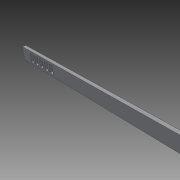
# Autodesk Inventor part: front_pane_middle
Saved by Autodesk Inventor 2014 (Build 180170000, 170)
## iProperties
Created: 2014-03-23
Part Number: front_pane_middle
Material: Generic
Document SubType Name: Modeling
Designer: buben
Density: 1 g/cm^3
Appearance: Default
Author: buben
Autodesk Inventor part; units mm, degrees
ref_plane "YZ Plane" through (0, 0, 0) normal (1, 0, 0) x (0, 1, 0)
ref_plane "XZ Plane" through (0, 0, 0) normal (0, 1, 0) x (-1, 0, 0)
ref_plane "XY Plane" through (0, 0, 0) normal (0, 0, 1) x (1, 0, 0)
sketch "Sketch1" plane through (0, 0, 0) normal (0, 1, 0) x (-1, 0, 0)
  line L0 (0, 0) -> (-300, 0)
  line L1 (-300, 0) -> (-300, -23.685)
  line L2 (-300, -23.685) -> (0, -23.685)
  line L3 (0, -23.685) -> (0, 0)
  dimension "d0" = 300
  dimension "d1" = 23.685
  constraints: 8 end point, 2 parallel, 1 horizontal, 1 perpendicular
  measures "d0" distance of L0.start L0.end
  measures "d1" distance of L2.end L0.start
extrude "Extrusion1" add sketch "Sketch1" along normal blind 6.5
sketch "Sketch2" plane through (0, 6.5, 0) normal (0, 1, 0) x (1, 0, 0)
  line L0 (0, 23.685) -> (0, 0) projected
  line L1 (21, 19.3425) -> (27, 19.3425)
  line L2 (28, 18.3425) -> (28, 5.3425)
  line L3 (27, 4.3425) -> (21, 4.3425)
  line L4 (20, 5.3425) -> (20, 18.3425)
  arc A0 (21, 19.3425) -> (20, 18.3425) centre (21, 18.3425) ccw
  arc A1 (20, 5.3425) -> (21, 4.3425) centre (21, 5.3425) ccw
  arc A2 (27, 4.3425) -> (28, 5.3425) centre (27, 5.3425) ccw
  arc A3 (28, 18.3425) -> (27, 19.3425) centre (27, 18.3425) ccw
  point P0 (20, 11.8425)
  point P1 (0, 11.8425)
  dimension "d4" = 1
  dimension "d5" = 15
  dimension "d6" = 8
  dimension "d7" = 20
  constraints: 8 end point, 8 point on circle, 8 tangent, 4 centre point, 3 equal radius, 2 midpoint, 2 parallel, 1 horizontal, 1 horizontal alignment, 1 perpendicular
  measures "d4" radius of A0
  measures "d5" distance between parallel lines of L3 L1
  measures "d6" distance between parallel lines of L2 L4
  measures "d7" distance between parallel lines of L0 L4
extrude "Extrusion2" cut sketch "Sketch2" against normal through all
pattern_linear "Rectangular Pattern1" count 5 spacing 12 along (1, 0, 0) of "Extrusion2"
body "Solid1"
